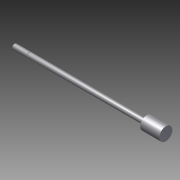
# Autodesk Inventor part: 0072-DXP0_rod
Saved by Autodesk Inventor 2012 (Build 160160000, 160)
## iProperties
Created: 2013-01-17
Part Number: 0072-DXP0_rod
Material: Default
Catalog Web Link: www.cadenas.de
Description: Standard Air Cylinder_rod-Original Line - Standard Air Cylinders
Vendor: BIMBA
Document SubType Name: Modeling
Designer: William
Manufacturer: BIMBA
Density: 1 g/cm^3
Category: PARTsolutions
Company: BIMBA
Title: 0072-DXP0_rod
Author: Cadenas PARTsolutions
Comments: Original Line - Standard Air Cylinders
PSOL_IDENT_0: {\\10.0.0.242\data_v9\23d-libs\bimba\bimba\bimba_imperial\bimba_full_line\original_line_cylinders\st
PSOL_IDENT_1: andard_air_cylinders\rod.prj},280 {VTYP=3D},{NB=0072-DXP0_rod},{LINA=0072-DXP0_rod},{NN=Standard Air
PSOL_IDENT_2: Cylinder_rod},{DATE=11.09.2012 07:37:40},{GEOMDATE=06.09.2012 09:06:00},{VERSION=},{LINEID=20},{LIN
PSOL_IDENT_3: ESUBID=-1},{WBVAR=STROKE,ACTING,MNT,DER,NR,BM,CO,M,EE,EEL,K,Q,Y,F,G,T,B,H,SER,SR,NT,W,E,HL,ST,STP,PR
PSOL_IDENT_4: C,PB,COLOR1}  {NB=0072-DXP0_rod},{LINA=0072-DXP0_rod},{KT=DUMMY},{PN=0072-DXP},{DASH=-},{BORE=0.3125
PSOL_IDENT_5: 0000},{BOREPN=007},{STROKE=2.000},{STROKEALG=[0.001:50/0.001]},{STROKE1=2.000},{ACTING=D},{ACTINGALG
PSOL_IDENT_6: = '' , 'Single Acting' , 'R' , 'Reverse Single Acting' , 'D' , 'Double Acting' },{ACTINGPN=D},{MNT=X
PSOL_IDENT_7: P},{MNTALG= '' , 'Front Nose Mounting' , 'XP' , 'Double End or Rear Pivot Mounting' , 'BF' , 'Front
PSOL_IDENT_8: Block Mounting' },{TYPE=},{MNTPN=XP},{DER=},{DERALG= '' , 'N/A' },{NR=},{NRALG= '' , 'N/A' },{NRPN=}
PSOL_IDENT_9: ,{BM=},{BMALG= '' , 'N/A' },{BMPN=},{CO=},{COALG= '' , 'N/A' },{M=},{MALG= '', 'Without Magnet', 'M'
PSOL_IDENT_10: , 'With Magnet' },{EE=},{EEL=0},{EEMAX=48},{EEALG= '', 'Without Extra Extension', 'EE', 'With Extra
PSOL_IDENT_11: Extension' },{EELALG=0},{EEPN=},{EEPN1=0.000},{K=},{KALG= '', 'Standard' , 'K' , 'Ports Rotated 90de
PSOL_IDENT_12: g' },{KPN=},{Q=},{QALG= '' , 'Without Side Ported Rear Head' , 'Q' , 'With Side Ported Rear Head' },
PSOL_IDENT_13: {QPN=},{Y=},{YALG= '' , 'With Pivot Bushing' },{YPN=},{F=},{FALG= '', 'Standard', 'F', 'Molycoated B
PSOL_IDENT_14: ody' },{FPN=},{G=},{GPN=},{T=},{TALG= '' , 'Standard' , 'N' , 'Low Temperature' , 'V' , 'High Temper
PSOL_IDENT_15: ature' },{NPN=},{VPN=},{B=},{BALG= '' , 'With Bumper' },{BPN=},{H=},{HALG= '', 'N/A' },{HPN=},{SER=}
PSOL_IDENT_16: ,{SERALG= '' , 'Without Spring Extend/Return' , 'JS' , 'With Spring Return' , 'JR' , 'With Spring Ex
PSOL_IDENT_17: tend' },{SR=},{SRALG= 'C' , 'Carbon Steel Rod' , 'SR' , '303 Stainless Steel Rod' , '' , '303 Stainl
PSOL_IDENT_18: ess Steel Rod1' },{SRPN=},{SRCON=0},{NT=},{NTPN=},{W=},{WALG= '' , 'Without Wiper' , 'W' , 'With Wip
PSOL_IDENT_19: er' },{WPN=},{E=},{EALG= '' , 'Without Special Lube and Seals' , 'E' , 'With Special Lube and Seals'
PSOL_IDENT_20: },{EPN=},{HL=},{HLALG= '' , 'Wihout Low Pressure Hydraulic' , 'HL' , 'With Low Pressure Hydraulic'
PSOL_IDENT_21: },{ST=},{STALG= '' , 'Without Switch Track' , 'T' , 'With Switch Track' },{STP=},{STPALG= '' , 'N/A'
PSOL_IDENT_22: },{STPN=},{PRC=},{PRCALG= '' , 'Without Piston Rod Clevis' , 'D-166-1' , 'With Piston Rod Clevis' }
PSOL_IDENT_23: ,{PRCPN=},{PB=},{PBALG= '' , 'Without Pivot Bracket' , 'D-167' , 'With Pivot Bracket' },{PBPN=},{TLE
PSOL_IDENT_24: N=2.7390},{TEXT=0.233333},{SPACE=0.133333},{FRAC=10.0300},{RGCON=},{RGDACCON=R},{RHCON=P},{RHCONON=1
PSOL_IDENT_25: },{RHACCON=R},{FNUTCON=1},{RNUTCON=0},{FNUTPN=D-344},{RNUTPN=D-801},{FNUTTRANS=0.0000},{RNUTTRANS=0.
PSOL_IDENT_26: 0000},{VHOLECON=0},{A1=0.8450},{A1N=0.6250},{A1P=0.8450},{A1B=0.9060},{A4=0.1585},{A4N=0.2550},{A4P=
PSOL_IDENT_27: 0.1585},{A5=0.0220},{A1H=0.875},{A1NH=0.3280},{A1PH=0.8750},{A1BH=0.0000},{A1SH=0.0000},{A2H=0.1585}
PSOL_IDENT_28: ,{A2NH=0.1585},{LENGTH=2.0300},{LENGTH1=2.0300},{LENGTH2=2.0400},{MUL=2.0000},{MUL11=2.0000},{MUL22=
PSOL_IDENT_29: 5.0000},{MUL33=3.0000},{MUL2=2.0000},{MUL211=2.0000},{MUL222=1.2500},{MUL233=0.7500},{SSS=4.0000},{R
PSOL_IDENT_30: GLEN=0.7085},{RHLEN=0.5825},{SSS1=4.0000},{A13=0.7190},{THDLEN1=0.3800},{THD1=0.1250},{TAB=UNC},{THD
PSOL_IDENT_31: LEN=0.3800},{THD=0.1250},{OD=0.3215},{RODL=3.6910},{PL=0.4660},{RODDIA=0.1250},{HEX=0.0000},{RODTRAN
PSOL_IDENT_32: S=0.0000},{G1=0.0000},{ON=0},{G5=0.0000},{DERLEN=3.2250},{THOLE=0.0000},{WF=0.0000},{BADD=0.0000},{M
PSOL_IDENT_33: ADD=0.0000},{NVADD=0.000},{JRADD=0.00000},{COLOR=0.71,0.71,0.71,0.00},{GROOVE=1},{HOL=0},{D7=0.1270}
PSOL_IDENT_34: ,{H1=0.0000},{D1=0.6050},{D1RH=0.4380},{D1P=0.0000},{D1B=0.6050},{D1N=0.3590},{D1NRH=0.3590},{D1BRH=
PSOL_IDENT_35: 0.0000},{D1PRH=0.4380},{BOZO=1},{HADD=0.000},{COLOR1=0},{DEFL=0.0000},{HEXL=0.0000},{SSADD=0.0000},{
PSOL_IDENT_36: WFL=0.0000},{MOVE=0.0000}
CNS_NT: Standard
CNS_NB: 0072-DXP0_rod
CNS_NBSYN: $PN.$COLOR1._rod
CNS_LINA: 0072-DXP0_rod
CNS_PN: 0072-DXP
CNS_DASH: -
CNS_BORE: 0.31250000
CNS_BOREPN: 007
CNS_STROKE: 2.000
CNS_STROKEALG: [0.001:50/0.001]
CNS_STROKE1: 2.000
CNS_ACTING: Double Acting
CNS_ACTINGALG: '' , 'Single Acting' , 'R' , 'Reverse Single Acting' , 'D' , 'Double Acting'
CNS_ACTINGPN: D
CNS_MNT: Double End or Rear Pivot Mounting
CNS_MNTALG: '' , 'Front Nose Mounting' , 'XP' , 'Double End or Rear Pivot Mounting' , 'BF' , 'Front Block Mounting'
CNS_MNTPN: XP
CNS_DER: N/A
CNS_DERALG: '' , 'N/A'
CNS_NR: N/A
CNS_NRALG: '' , 'N/A'
CNS_BM: N/A
CNS_BMALG: '' , 'N/A'
CNS_CO: N/A
CNS_COALG: '' , 'N/A'
CNS_M: Without Magnet
CNS_MALG: '', 'Without Magnet', 'M', 'With Magnet'
CNS_EE: Without Extra Extension
CNS_EEL: 0
CNS_EEMAX: 48
CNS_EEALG: '', 'Without Extra Extension', 'EE', 'With Extra Extension'
CNS_EELALG: 0
CNS_EEPN1: 0.000
CNS_K: Standard
CNS_KALG: '', 'Standard' , 'K' , 'Ports Rotated 90deg'
CNS_Q: Without Side Ported Rear Head
CNS_QALG: '' , 'Without Side Ported Rear Head' , 'Q' , 'With Side Ported Rear Head'
CNS_Y: With Pivot Bushing
CNS_YALG: '' , 'With Pivot Bushing'
CNS_F: Standard
CNS_FALG: '', 'Standard', 'F', 'Molycoated Body'
CNS_G: Without Magnalube Lubrication
CNS_T: Standard
CNS_TALG: '' , 'Standard' , 'N' , 'Low Temperature' , 'V' , 'High Temperature'
CNS_B: With Bumper
CNS_BALG: '' , 'With Bumper'
CNS_H: N/A
CNS_HALG: '', 'N/A'
CNS_SER: Without Spring Extend/Return
CNS_SERALG: '' , 'Without Spring Extend/Return' , 'JS' , 'With Spring Return' , 'JR' , 'With Spring Extend'
CNS_SR: 303 Stainless Steel Rod1
CNS_SRALG: 'C' , 'Carbon Steel Rod' , 'SR' , '303 Stainless Steel Rod' , '' , '303 Stainless Steel Rod1'
CNS_SRCON: 0
CNS_W: Without Wiper
CNS_WALG: '' , 'Without Wiper' , 'W' , 'With Wiper'
CNS_E: Without Special Lube and Seals
CNS_EALG: '' , 'Without Special Lube and Seals' , 'E' , 'With Special Lube and Seals'
CNS_HL: Wihout Low Pressure Hydraulic
CNS_HLALG: '' , 'Wihout Low Pressure Hydraulic' , 'HL' , 'With Low Pressure Hydraulic'
CNS_ST: Without Switch Track
CNS_STALG: '' , 'Without Switch Track' , 'T' , 'With Switch Track'
CNS_STP: N/A
CNS_STPALG: '' , 'N/A'
CNS_PRC: Without Piston Rod Clevis
CNS_PRCALG: '' , 'Without Piston Rod Clevis' , 'D-166-1' , 'With Piston Rod Clevis'
CNS_PB: Without Pivot Bracket
CNS_PBALG: '' , 'Without Pivot Bracket' , 'D-167' , 'With Pivot Bracket'
CNS_TLEN: 2.7390
CNS_TEXT: 0.233
CNS_SPACE: 0.133
CNS_FRAC: 10.0300
CNS_RGDACCON: R
CNS_RHCON: P
CNS_RHCONON: 1
CNS_RHACCON: R
CNS_FNUTCON: 1
CNS_RNUTCON: 0
CNS_FNUTPN: D-344
CNS_RNUTPN: D-801
CNS_FNUTTRANS: 0.0000
CNS_RNUTTRANS: 0.0000
CNS_VHOLECON: 0
CNS_A1: 0.8450
CNS_A1N: 0.6250
CNS_A1P: 0.8450
CNS_A1B: 0.9060
CNS_A4: 0.1585
CNS_A4N: 0.2550
CNS_A4P: 0.1585
CNS_A5: 0.0220
CNS_A1H: 0.875
CNS_A1NH: 0.3280
CNS_A1PH: 0.8750
CNS_A1BH: 0.0000
CNS_A1SH: 0.0000
CNS_A2H: 0.1585
CNS_A2NH: 0.1585
CNS_LENGTH: 2.0300
CNS_LENGTH1: 2.0300
CNS_LENGTH2: 2.0400
CNS_MUL: 2.0000
CNS_MUL11: 2.0000
CNS_MUL22: 5.0000
CNS_MUL33: 3.0000
CNS_MUL2: 2.0000
CNS_MUL211: 2.0000
CNS_MUL222: 1.2500
CNS_MUL233: 0.7500
CNS_SSS: 4.0000
CNS_RGLEN: 0.7085
CNS_RHLEN: 0.5825
CNS_SSS1: 4.0000
CNS_A13: 0.7190
CNS_THDLEN1: 0.3800
CNS_THD1: 0.1250
CNS_TAB: UNC
CNS_THDLEN: 0.3800
CNS_THD: 0.1250
CNS_OD: 0.3215
CNS_RODL: 3.6910
CNS_PL: 0.4660
CNS_RODDIA: 0.1250
CNS_HEX: 0.0000
CNS_RODTRANS: 0.0000
CNS_G1: 0.0000
CNS_ON: 0
CNS_G5: 0.0000
CNS_DERLEN: 3.2250
CNS_THOLE: 0.0000
CNS_WF: 0.0000
CNS_BADD: 0.0000
CNS_MADD: 0.0000
CNS_NVADD: 0.000
CNS_JRADD: 0.00000
CNS_COLOR: 0.71,0.71,0.71,0.00
CNS_GROOVE: 1
CNS_HOL: 0
CNS_D7: 0.1270
CNS_H1: 0.0000
CNS_D1: 0.6050
CNS_D1RH: 0.4380
CNS_D1P: 0.0000
CNS_D1B: 0.6050
CNS_D1N: 0.3590
CNS_D1NRH: 0.3590
CNS_D1BRH: 0.0000
CNS_D1PRH: 0.4380
CNS_BOZO: 1
CNS_HADD: 0.000
CNS_COLOR1: 0
CNS_DEFL: 0.0000
CNS_HEXL: 0.0000
CNS_SSADD: 0.0000
CNS_WFL: 0.0000
CNS_MOVE: 0.0000
SUPPLIER: BIMBA
ARTICLENO: 0072-DXP0_rod
BOMINFO: 0072-DXP0_rod
CREATOR: CADENAS GmbH
Autodesk Inventor part; units mm, degrees
sketch "Sketch_1" plane through (0, 0, 0) normal (0, 0, 1) x (1, 0, 0)
  line L0 (84.0994, 0) -> (0, 0)
  line L1 (0, 0) -> (0, 1.5875)
  line L2 (0, 1.5875) -> (72.263, 1.5875)
  line L3 (72.263, 1.5875) -> (72.263, 4.0323)
  line L4 (72.263, 4.0323) -> (84.0994, 4.0323)
  line L5 (84.0994, 4.0323) -> (84.0994, 0)
  line L6 (84.0994, 0) -> (0, 0)
  constraints: 14 end point
revolve "Revolution1" add sketch "Sketch_1" angle 360 about axis through (84.0994, 0, 0) along (1, 0, 0)
sketch "Sketch_2" plane through (0, 0, 0) normal (0, 0, 1) x (1, 0, 0)
  line L0 (0, 0) -> (-9.652, 0)
  line L1 (-9.652, 0) -> (-9.652, 1.209)
  line L2 (-9.652, 1.209) -> (-9.2735, 1.5875)
  line L3 (-9.2735, 1.5875) -> (0, 1.5875)
  line L4 (0, 1.5875) -> (0, 0)
  line L5 (0, 0) -> (-9.652, 0)
  constraints: 12 end point
revolve "Revolution2" add sketch "Sketch_2" angle 360 about axis through (0, 0, 0) along (1, 0, 0)
sketch "Sketch_30" plane through (0, 0, 0) normal (0, 0, 1) x (1, 0, 0)
  line L0 (0, 0) -> (-0.254, 0)
  line L1 (-0.254, 1.8415) -> (-0.254, 1.3335)
  line L2 (-0.254, 1.3335) -> (0, 1.3335)
  line L3 (0, 1.3335) -> (0, 1.8415)
  line L4 (0, 1.8415) -> (-0.254, 1.8415)
  constraints: 10 end point
revolve "Revolution3" cut sketch "Sketch_30" angle 360 about axis through (0, 0, 0) along (1, 0, 0)
ref_plane "rod_cp_XY" through (0, 0, 0) normal (1, 0, 0) x (0, 0, -1)
ref_plane "rod_cp_YZ" through (0, 0, 0) normal (0, 0, -1) x (0, 1, 0)
ref_plane "rod_cp_ZX" through (0, 0, 0) normal (0, 1, 0) x (1, 0, 0)
ref_plane "to_rod_clevis_XY" through (-9.652, 0, 0) normal (1, 0, 0) x (0, 0, -1)
ref_plane "to_rod_clevis_YZ" through (-9.652, 0, 0) normal (0, 0, -1) x (0, 1, 0)
ref_plane "to_rod_clevis_ZX" through (-9.652, 0, 0) normal (0, 1, 0) x (1, 0, 0)
ref_plane "rl2_XY" through (0, 0, 0) normal (1, 0, 0) x (0, 0, -1)
ref_plane "rl2_YZ" through (0, 0, 0) normal (0, 0, -1) x (0, 1, 0)
ref_plane "rl2_ZX" through (0, 0, 0) normal (0, 1, 0) x (1, 0, 0)
ref_plane "rl1_XY" through (-9.652, 0, 0) normal (1, 0, 0) x (0, 0, -1)
ref_plane "rl1_YZ" through (-9.652, 0, 0) normal (0, 0, -1) x (0, 1, 0)
ref_plane "rl1_ZX" through (-9.652, 0, 0) normal (0, 1, 0) x (1, 0, 0)
ref_plane "thd1_XY" through (-9.652, 1.5875, 0) normal (1, 0, 0) x (0, 0, -1)
ref_plane "thd1_YZ" through (-9.652, 1.5875, 0) normal (0, 0, -1) x (0, 1, 0)
ref_plane "thd1_ZX" through (-9.652, 1.5875, 0) normal (0, 1, 0) x (1, 0, 0)
ref_plane "thd2_XY" through (-9.652, -1.5875, 0) normal (1, 0, 0) x (0, 0, -1)
ref_plane "thd2_YZ" through (-9.652, -1.5875, 0) normal (0, 0, -1) x (0, 1, 0)
ref_plane "thd2_ZX" through (-9.652, -1.5875, 0) normal (0, 1, 0) x (1, 0, 0)
ref_plane "dia1_XY" through (0, 1.5875, 0) normal (1, 0, 0) x (0, 0, -1)
ref_plane "dia1_YZ" through (0, 1.5875, 0) normal (0, 0, -1) x (0, 1, 0)
ref_plane "dia1_ZX" through (0, 1.5875, 0) normal (0, 1, 0) x (1, 0, 0)
ref_plane "dia2_XY" through (0, -1.5875, 0) normal (1, 0, 0) x (0, 0, -1)
ref_plane "dia2_YZ" through (0, -1.5875, 0) normal (0, 0, -1) x (0, 1, 0)
ref_plane "dia2_ZX" through (0, -1.5875, 0) normal (0, 1, 0) x (1, 0, 0)
ref_plane "dia1r_XY" through (0, 0, 5.5626) normal (1, 0, 0) x (0, 0, -1)
ref_plane "dia1r_YZ" through (0, 0, 5.5626) normal (0, 0, -1) x (0, 1, 0)
ref_plane "dia1r_ZX" through (0, 0, 5.5626) normal (0, 1, 0) x (1, 0, 0)
ref_plane "dia2r_XY" through (0, 0, -5.5626) normal (1, 0, 0) x (0, 0, -1)
ref_plane "dia2r_YZ" through (0, 0, -5.5626) normal (0, 0, -1) x (0, 1, 0)
ref_plane "dia2r_ZX" through (0, 0, -5.5626) normal (0, 1, 0) x (1, 0, 0)
ref_plane "dia12_XY" through (0, 0, 7.6835) normal (1, 0, 0) x (0, 0, -1)
ref_plane "dia12_YZ" through (0, 0, 7.6835) normal (0, 0, -1) x (0, 1, 0)
ref_plane "dia12_ZX" through (0, 0, 7.6835) normal (0, 1, 0) x (1, 0, 0)
ref_plane "dia22_XY" through (0, 0, -7.6835) normal (1, 0, 0) x (0, 0, -1)
ref_plane "dia22_YZ" through (0, 0, -7.6835) normal (0, 0, -1) x (0, 1, 0)
ref_plane "dia22_ZX" through (0, 0, -7.6835) normal (0, 1, 0) x (1, 0, 0)
body "Solid1"
